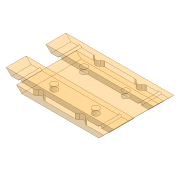
# Autodesk Inventor part: flange7-42mm
Saved by Autodesk Inventor 2021 (Build 250183000, 183)
## iProperties
Created: 2022-10-18
Part Number: flange7-42mm
Material: Rubber, Silicone
Document SubType Name: Modeling
Designer: alyn649
Density: 1.25 g/cm^3
Appearance: Clear - Yellow(1)
Author: alyn649
Autodesk Inventor part; units mm, degrees
ref_plane "YZ Plane" through (0, 0, 0) normal (1, 0, 0) x (0, 1, 0)
ref_plane "XZ Plane" through (0, 0, 0) normal (0, 1, 0) x (-1, 0, 0)
ref_plane "XY Plane" through (0, 0, 0) normal (0, 0, 1) x (1, 0, 0)
sketch "Sketch2" plane through (0, 0, 0) normal (0, 0, 1) x (1, 0, 0)
  line L0 (-13.18, 0) -> (13.18, 0)
  line L1 (13.18, 0) -> (11.6267, -1.5)
  line L2 (11.6267, -1.5) -> (-11.6267, -1.5)
  line L3 (-11.6267, -1.5) -> (-13.18, 0)
  line L4 (-8.8153, 7.7377) -> (-16.0231, 7.7377) construction
  line L5 (13.18, 0) -> (19.7494, 0) construction
  point P0 (0, 0)
  point P1 (0, 0)
  dimension "d0" = 26.36
  dimension "d1" = 136
  dimension "d2" = 136
  dimension "d3" = 1.5
  constraints: 12 end point, 3 horizontal, 1 coincident, 1 midpoint, 1 parallel
  measures "d0" distance of L0.start L0.end
  measures "d1" angle of L3 L4
  measures "d2" angle of L5 L1
  measures "d3" distance between parallel lines of L0 L2
extrude "Extrusion1" add sketch "Sketch2" along normal mid plane 18
sketch "Sketch3" plane through (-13.18, 0, 9) normal (0, 1, 0) x (1, 0, 0)
  circle A0 centre (6.893, 13.5) radius 1
  line L0 (0, 18) -> (26.36, 18) construction
  circle A1 centre (6.893, 18) radius 1 construction
  arc A2 (6.027, 17.5) -> (5.1609, 18) centre (5.1609, 17) ccw
  arc A3 (6.027, 17.5) -> (7.759, 17.5) centre (6.893, 18) ccw
  arc A4 (8.6251, 18) -> (7.759, 17.5) centre (8.6251, 17) ccw
  line L1 (5.1609, 18) -> (8.6251, 18)
  point P0 (13.18, 9)
  dimension "d6" = 6.287
  dimension "d7" = 4.5
  dimension "d8" = 2
  dimension "d9" = 2
  dimension "d10" = 1
  dimension "d11" = 1
  constraints: 8 point on circle, 7 tangent, 5 centre point, 4 point on line, 2 end point, 1 vertical alignment
  measures "d6" horizontal distance of A0.centre point (13.18, 9)
  measures "d7" vertical distance of A0.centre point (13.18, 9)
  measures "d8" diameter of A1
  measures "d9" diameter of A0
  measures "d10" radius of A2
  measures "d11" radius of A4
extrude "Extrusion2" add sketch "Sketch3" along normal blind 1.5
mirror "Mirror2" about plane through (0, 0, 0) normal (1, 0, 0) of "Extrusion2"
mirror "Mirror3" about plane through (0, 0, 0) normal (0, 0, 1) of "Extrusion2", "Mirror2"
sketch "Sketch4" plane through (-6.287, 1.5, 4.5) normal (0, 1, 0) x (1, 0, 0)
  line L0 (-11.213, 1.5) -> (23.787, 1.5)
  line L1 (23.787, 1.5) -> (23.787, -4.5)
  line L2 (23.787, -4.5) -> (-11.213, -4.5)
  line L3 (-11.213, -4.5) -> (-11.213, 1.5)
  line L4 (10.8419, -4.5) -> (1.7321, -4.5) construction
  circle A0 centre (0, 0) radius 1 construction
  line L5 (3.7226, 1) -> (2.6401, 1) construction
  point P0 (6.287, 4.5)
  point P1 (6.287, -4.5)
  dimension "d15" = 0.5
  dimension "d16" = 35
  constraints: 10 end point, 2 horizontal, 2 midpoint, 2 parallel, 1 perpendicular, 1 tangent
  measures "d15" distance between parallel lines of L0 L5
  measures "d16" distance between parallel lines of L1 L3
extrude "Extrusion3" add sketch "Sketch4" along normal blind 1.5
mirror "Mirror4" about plane through (0, 0, 0) normal (0, 0, 1) of "Extrusion3"
sketch "Sketch5" plane through (0, 0, 9) normal (0, 0, 1) x (1, 0, 0)
  line L0 (-13.18, 0) -> (-11.6267, -1.5) projected
  line L1 (-8.0191, 0) -> (-13.18, 0) projected
  line L2 (-13.18, 0) -> (-18.1793, 4.8277)
  line L3 (-17.5371, 6.2929) -> (-7.2761, -3.6161) construction
  circle A0 centre (-12.074, 1.5) radius 0.5
  line L4 (-17.5, 1.5) -> (-8.0191, 1.5) projected
  line L5 (-18.1793, 4.8277) -> (-18.1793, 0)
  line L6 (-18.1793, 0) -> (-13.18, 0)
  point P0 (0, 0)
  point P1 (-12.574, 1.5)
  point P2 (-11.574, 1.5)
  dimension "d20" = 1
  dimension "d19" = 1.5
  constraints: 8 end point, 3 point on line, 1 collinear, 1 parallel, 1 perpendicular, 1 vertical, 3 other
  measures "d19" distance between parallel lines of L3 L2
extrude "Extrusion4" cut sketch "Sketch5" against normal through all contours L6 L5 L2 | L4 A0 picked at (-12.0539, 1.6655)
mirror "Mirror5" about plane through (0, 0, 0) normal (1, 0, 0) of "Extrusion4"
equation "\"d2\" = d1"
equation "\"d11\" = d10"
body "Solid1"
